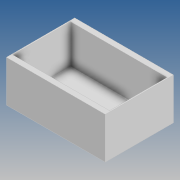
# Autodesk Inventor part: aluminium_project_box
Saved by Autodesk Inventor 2020 (Build 240168000, 168)
## iProperties
Created: 2021-04-15
Part Number: aluminium_project_box
Material: Generic
Document SubType Name: Modeling
Designer: stephen
Density: 1 g/cm^3
Appearance: Default
Author: stephen
Autodesk Inventor part; units mm, degrees
ref_plane "YZ Plane" through (0, 0, 0) normal (1, 0, 0) x (0, 1, 0)
ref_plane "XZ Plane" through (0, 0, 0) normal (0, 1, 0) x (-1, 0, 0)
ref_plane "XY Plane" through (0, 0, 0) normal (0, 0, 1) x (1, 0, 0)
sketch "Sketch1" plane through (0, 0, 0) normal (0, 1, 0) x (-1, 0, 0)
  line L0 (-54.991, 37.973) -> (54.991, 37.973)
  line L1 (54.991, 37.973) -> (54.991, -37.973)
  line L2 (54.991, -37.973) -> (-54.991, -37.973)
  line L3 (-54.991, -37.973) -> (-54.991, 37.973)
  line L4 (-54.991, 37.973) -> (54.991, -37.973) construction
  line L5 (54.991, 37.973) -> (-54.991, -37.973) construction
  point P0 (0, 0)
  dimension "d0" = 109.982
  dimension "d1" = 75.946
  constraints: 12 end point, 2 midpoint, 2 parallel, 1 horizontal, 1 perpendicular
  measures "d0" distance of L0.start L0.end
  measures "d1" distance of L0.end L1.end
extrude "Extrusion1" add sketch "Sketch1" along normal blind 45.974
sketch "Sketch2" plane through (0, 45.974, 0) normal (0, 1, 0) x (1, 0, 0)
  line L0 (53.721, -32.004) -> (-53.721, -32.004)
  line L1 (-53.721, -32.004) -> (-53.721, 32.004)
  line L2 (-53.721, 32.004) -> (53.721, 32.004)
  line L3 (53.721, 32.004) -> (53.721, -32.004)
  line L4 (53.721, -32.004) -> (-53.721, 32.004) construction
  line L5 (-53.721, -32.004) -> (53.721, 32.004) construction
  line L6 (-54.991, 37.973) -> (-54.991, -37.973) projected
  point P0 (0, 0)
  dimension "d4" = 1.27
  dimension "d5" = 64.008
  constraints: 12 end point, 2 midpoint, 2 parallel, 1 horizontal, 1 perpendicular
  measures "d4" distance between parallel lines of L1 L6
  measures "d5" distance between parallel lines of L0 L2
extrude "Extrusion2" cut sketch "Sketch2" against normal blind 42.926
body "Solid1"
